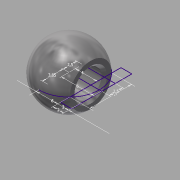
# Autodesk Inventor part: KULA
Saved by Autodesk Inventor 2013 (Build 170138000, 138)
## iProperties
Created: 2015-04-17
Part Number: KULA
Material: Stainless Steel
Document SubType Name: Modeling
Designer: Ultimate
Density: 1 g/cm^3
Author: Ultimate
Autodesk Inventor part; units mm, degrees
ref_plane "YZ Plane" through (0, 0, 0) normal (1, 0, 0) x (0, 1, 0)
ref_plane "XZ Plane" through (0, 0, 0) normal (0, 1, 0) x (-1, 0, 0)
ref_plane "XY Plane" through (0, 0, 0) normal (0, 0, 1) x (1, 0, 0)
sketch "Sketch1" plane through (0, 0, 0) normal (0, 0, 1) x (1, 0, 0)
  line L0 (0, 3.85) -> (0, -3.85)
  line L1 (0, -3.85) -> (4, -3.85)
  line L2 (4, -3.85) -> (4, 3.85)
  line L3 (4, 3.85) -> (0, 3.85)
  arc A0 (0, -5.5518) -> (0, 5.5518) centre (0, 0) ccw
  line L4 (0, 5.5518) -> (0, -5.5518)
  line L5 (4, 5.5518) -> (6, 5.5518)
  line L6 (6, 5.5518) -> (6, -5.5518)
  line L7 (6, -5.5518) -> (4, -5.5518)
  line L8 (4, -5.5518) -> (4, 5.5518)
  line L9 (0, 2.5) -> (6, 2.5)
  line L10 (6, 2.5) -> (6, 0)
  line L11 (6, 0) -> (0, 0)
  line L12 (0, 0) -> (0, 2.5)
  dimension "d0" = 7.7
  dimension "d2" = 4
  dimension "d3" = 3.85
  dimension "d4" = 2
  dimension "d5" = 2
  dimension "d6" = 6
  dimension "d7" = 6
  dimension "d8" = 2.5
  dimension "d9" = 2.5
  constraints: 26 end point, 6 parallel, 4 perpendicular, 3 point on circle, 2 horizontal, 2 tangent, 1 centre point, 1 coincident, 1 midpoint, 1 point on line, 1 vertical
  measures "d0" distance of L1.end L2.end
  measures "d2" distance from line of point (0, 0) L2
  measures "d3" distance from line of L1 point (0, 0)
  measures "d4" distance of L6.end L7.end
  measures "d5" distance between parallel lines of L6 L2
  measures "d6" distance between parallel lines of L6 L4
  measures "d7" distance of L10.end L11.end
  measures "d8" distance of L9.end L10.end
  measures "d9" distance from line of L9 point (0, 0)
revolve "Revolution1" add sketch "Sketch1" angle 360 about axis through (0, 5.5518, 0) along (0, -1, 0) contours L3 L2 L9 L0 | L4 A0 L3 | L9 L2 L11 L0 | A0 L9 L2 | L11 L2 L1 L0 | L9 A0 L11 L2 | L1 A0 L4 | L11 A0 L2
extrude "Extrusion1" cut sketch "Sketch1" along normal mid plane 10 contours A0 L9 L2 | L8 L5 L6 L9 A0 | L9 A0 L11 L2 | L9 L6 L11 A0 | L11 A0 L2 | L11 L6 L7 L8 A0
mirror "Mirror1" about plane through (0, 0, 0) normal (1, 0, 0) of "Extrusion1"
revolve "Revolution2" cut sketch "Sketch1" angle 360 about axis through (6, 0, 0) along (-1, 0, 0) contours L9 L2 L11 L0 | L9 A0 L11 L2 | L9 L6 L11 A0
mirror "Mirror2" about plane through (0, 1.25, 0) normal (1, 0, 0) of "Revolution2"
chamfer "Chamfer1" distance 0.5 angle 45 2 edges at (-4, -2.5, 0) (4, -2.5, 0)
body "Solid1"
